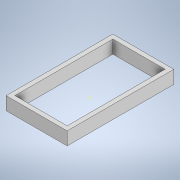
# Autodesk Inventor part: servo_holder
Saved by Autodesk Inventor 2021 (Build 250183000, 183)
## iProperties
Created: 2024-05-23
Part Number: servo_holder
Material: Generic
Document SubType Name: Modeling
Designer: 23adrdam
Density: 1 g/cm^3
Appearance: Default
Author: 23adrdam
Autodesk Inventor part; units mm, degrees
ref_plane "YZ Plane" through (0, 0, 0) normal (1, 0, 0) x (0, 1, 0)
ref_plane "XZ Plane" through (0, 0, 0) normal (0, 1, 0) x (-1, 0, 0)
ref_plane "XY Plane" through (0, 0, 0) normal (0, 0, 1) x (1, 0, 0)
sketch "Sketch1" plane through (0, 0, 0) normal (0, 1, 0) x (-1, 0, 0)
  point P0 (0, 0)
sketch "Sketch2" plane through (0, 0, 0) normal (0, 1, 0) x (-1, 0, 0)
  line L0 (-6.005, -11.25) -> (6.005, -11.25)
  line L1 (6.005, -11.25) -> (6.005, 11.25)
  line L2 (6.005, 11.25) -> (-6.005, 11.25)
  line L3 (-6.005, 11.25) -> (-6.005, -11.25)
  line L4 (-6.005, -11.25) -> (6.005, 11.25) construction
  line L5 (6.005, -11.25) -> (-6.005, 11.25) construction
  line L6 (-7.005, -12.25) -> (7.005, -12.25)
  line L7 (7.005, -12.25) -> (7.005, 12.25)
  line L8 (7.005, 12.25) -> (-7.005, 12.25)
  line L9 (-7.005, 12.25) -> (-7.005, -12.25)
  line L10 (-7.005, -12.25) -> (7.005, 12.25) construction
  line L11 (7.005, -12.25) -> (-7.005, 12.25) construction
  point P0 (0, 0)
  dimension "d0" = 22.5
  dimension "d1" = 12.01
  dimension "d2" = 24.5
  dimension "d3" = 14.01
  constraints: 24 end point, 4 midpoint, 4 parallel, 2 horizontal, 2 perpendicular
  measures "d0" distance of L0.end L1.end
  measures "d1" distance of L1.end L2.end
  measures "d2" distance of L6.end L7.end
  measures "d3" distance of L7.end L8.end
extrude "Extrusion1" add sketch "Sketch2" along normal blind 3
body "Solid1"
